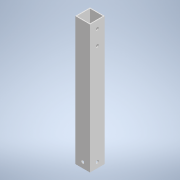
# Autodesk Inventor part: metal tube piece
Saved by Autodesk Inventor 2020.1 (Build 241239000, 239)
## iProperties
Created: 2019-11-07
Part Number: metal tube piece
Material: Generic
Document SubType Name: Modeling
Designer: amirs
Density: 1 g/cm^3
Appearance: Default
Author: amirs
Autodesk Inventor part; units mm, degrees
ref_plane "YZ Plane" through (0, 0, 0) normal (1, 0, 0) x (0, 1, 0)
ref_plane "XZ Plane" through (0, 0, 0) normal (0, 1, 0) x (-1, 0, 0)
ref_plane "XY Plane" through (0, 0, 0) normal (0, 0, 1) x (1, 0, 0)
sketch "Sketch1" plane through (0, 0, 0) normal (0, 1, 0) x (-1, 0, 0)
  line L0 (-12.7, 12.7) -> (12.7, 12.7)
  line L1 (12.7, 12.7) -> (12.7, -12.7)
  line L2 (12.7, -12.7) -> (-12.7, -12.7)
  line L3 (-12.7, -12.7) -> (-12.7, 12.7)
  line L4 (-12.7, 12.7) -> (12.7, -12.7) construction
  line L5 (12.7, 12.7) -> (-12.7, -12.7) construction
  line L6 (11.1125, -11.1125) -> (11.1125, 11.1125)
  line L7 (11.1125, 11.1125) -> (-11.1125, 11.1125)
  line L8 (-11.1125, 11.1125) -> (-11.1125, -11.1125)
  line L9 (-11.1125, -11.1125) -> (11.1125, -11.1125)
  point P0 (0, 0)
  dimension "d0" = 25.4
  dimension "d1" = 25.4
  dimension "d2" = 1.5875
  constraints: 20 end point, 4 parallel, 2 midpoint, 2 perpendicular, 1 horizontal, 3 other
  measures "d0" distance of L1.end L2.end
  measures "d1" distance of L2.end L0.start
  measures "d2" distance between parallel lines of L1 L6
extrude "Extrusion1" add sketch "Sketch1" along normal blind 220.98
sketch "Sketch2" plane through (12.7, 0, 12.7) normal (1, 0, 0) x (0, 0, -1)
  line L0 (12.7, 0) -> (22.225, 0) construction
  line L1 (0, 0) -> (25.4, 0) construction
  line L2 (12.7, 0) -> (3.175, 0) construction
  line L3 (3.175, 0) -> (3.175, 19.05) construction
  line L4 (3.175, 19.05) -> (22.225, 19.05) construction
  line L5 (22.225, 19.05) -> (22.225, 0) construction
  line L6 (3.175, 19.05) -> (22.225, 0) construction
  line L7 (22.225, 19.05) -> (3.175, 0) construction
  circle A0 centre (12.7, 9.525) radius 2.4384
  dimension "d5" = 9.525
  dimension "d7" = 9.525
  dimension "d8" = 19.05
  dimension "d9" = 4.8768
  constraints: 14 end point, 3 perpendicular, 3 point on line, 1 centre point, 1 midpoint, 1 vertical
  measures "d5" distance of L0.start L0.end
  measures "d7" distance of L0.start L2.end
  measures "d8" distance of L2.end L3.end
  measures "d9" diameter of A0
extrude "Extrusion2" cut sketch "Sketch2" against normal blind 25.4
sketch "Sketch3" plane through (12.7, 0, -12.7) normal (0, 0, -1) x (-1, 0, 0)
  line L0 (12.7, 0) -> (22.225, 0) construction
  line L1 (0, 0) -> (25.4, 0) construction
  line L2 (12.7, 0) -> (3.175, 0) construction
  line L3 (3.175, 0) -> (3.175, 19.05) construction
  line L4 (3.175, 19.05) -> (22.225, 19.05) construction
  line L5 (22.225, 19.05) -> (22.225, 0) construction
  line L6 (3.175, 19.05) -> (22.225, 0) construction
  line L7 (22.225, 19.05) -> (3.175, 0) construction
  circle A0 centre (12.7, 9.525) radius 2.4384
  point P0 (12.7, 0)
  dimension "d13" = 9.525
  dimension "d14" = 9.525
  dimension "d15" = 19.05
  dimension "d16" = 4.8768
  constraints: 16 end point, 3 perpendicular, 3 point on line, 1 centre point, 1 midpoint, 1 vertical
  measures "d13" distance of L0.start L0.end
  measures "d14" distance of L0.start L2.end
  measures "d15" distance of L2.end L3.end
  measures "d16" diameter of A0
extrude "Extrusion3" cut sketch "Sketch3" against normal blind 25.4
sketch "Sketch4" plane through (12.7, 0, 12.7) normal (1, 0, 0) x (0, 0, -1)
  circle A0 centre (12.7, 208.28) radius 2.4384
  circle A1 centre (12.7, 182.88) radius 2.4384
  line L0 (0, 220.98) -> (25.4, 220.98) projected
  point P0 (12.7, 0)
  dimension "d19" = 12.7
  dimension "d20" = 4.8768
  dimension "d21" = 25.4
  constraints: 2 centre point, 2 vertical alignment, 1 equal radius
  measures "d19" distance from line of L0 A0.centre
  measures "d20" diameter of A1
  measures "d21" distance of A0.centre A1.centre
extrude "Extrusion4" cut sketch "Sketch4" against normal blind 7.62
equation "\"d7\" = d5"
equation "\"d14\" = d13"
body "Solid1"
